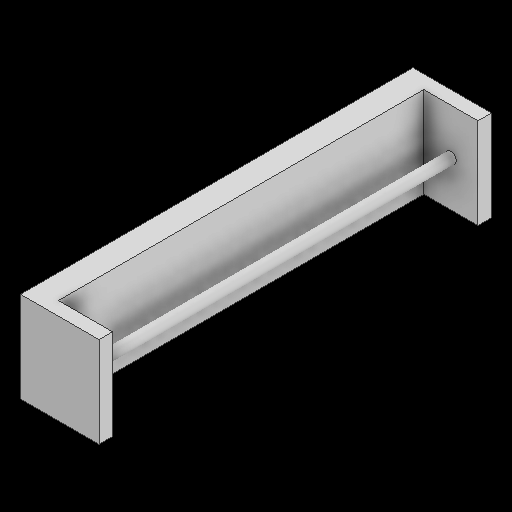
# Autodesk Inventor part: linear_motor
Saved by Autodesk Inventor 2025.1 (Build 291241000, 241)
## iProperties
Created: 2024-08-22
Part Number: linear_motor
Material: 일반
Document SubType Name: Modeling
Designer: ojs08
Density: 1 g/cm^3
Appearance: 기본값
Author: ojs08
Autodesk Inventor part; units mm, degrees
ref_plane "YZ Plane" through (0, 0, 0) normal (1, 0, 0) x (0, 1, 0)
ref_plane "XZ Plane" through (0, 0, 0) normal (0, 1, 0) x (-1, 0, 0)
ref_plane "XY Plane" through (0, 0, 0) normal (0, 0, 1) x (1, 0, 0)
sketch "스케치1" plane through (0, 0, 0) normal (0, 0, 1) x (1, 0, 0)
  line L0 (0, 0) -> (29, 0)
  line L1 (29, 0) -> (29, -33.5)
  line L2 (29, -33.5) -> (0, -33.5)
  line L3 (0, -33.5) -> (0, 0)
  dimension "d0" = 29
  dimension "d1" = 33.5
  constraints: 8 end point, 2 parallel, 1 coincident, 1 horizontal, 1 perpendicular
  measures "d0" distance of L0.start L0.end
  measures "d1" distance of L2.end L0.start
extrude "돌출1" add sketch "스케치1" along normal blind 145
sketch "스케치2" plane through (29, -33.5, 0) normal (1, 0, 0) x (0, 0, -1)
  line L0 (0, 0) -> (0, 33.5) projected
  line L1 (0, 33.5) -> (-145, 33.5) projected
  line L2 (-145, 0) -> (-145, 33.5) projected
  line L3 (0, 0) -> (-145, 0) projected
  line L4 (-140, 33.5) -> (-140, 0)
  line L5 (-5, 33.5) -> (-5, 0)
  dimension "d4" = 5
  dimension "d5" = 5
  constraints: 4 end point, 4 point on line, 2 perpendicular
  measures "d4" distance between parallel lines of L4 L2
  measures "d5" distance between parallel lines of L0 L5
extrude "돌출2" cut sketch "스케치2" against normal blind 20 contours L3 L4 L1 L5
sketch "스케치3" plane through (29, -33.5, 140) normal (0, 0, -1) x (-1, 0, 0)
  line L0 (0, 0) -> (0, 33.5) projected
  line L1 (20, 0) -> (0, 0) projected
  line L2 (20, 0) -> (20, 33.5) projected
  line L3 (0, 33.5) -> (20, 33.5) projected
  circle A0 centre (10, 16.75) radius 2
  point P0 (29, 33.5)
  dimension "d8" = 4
  dimension "d9" = 10
  dimension "d10" = 16.75
  constraints: 1 centre point
  measures "d8" diameter of A0
  measures "d9" distance from line of L0 A0.centre
  measures "d10" distance from line of L1 A0.centre
extrude "돌출3" add sketch "스케치3" along normal up to surface (135 mm away) contours A0
